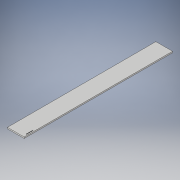
# Autodesk Inventor part: BBM
Saved by Autodesk Inventor 2019.4 (Build 234330000, 330)
## iProperties
Created: 2021-02-08
Part Number: BBM
Material: Generic
Document SubType Name: Modeling
Designer: caleb
Density: 1 g/cm^3
Appearance: Default
Author: caleb
Autodesk Inventor part; units mm, degrees
ref_plane "YZ Plane" through (0, 0, 0) normal (1, 0, 0) x (0, 1, 0)
ref_plane "XZ Plane" through (0, 0, 0) normal (0, 1, 0) x (-1, 0, 0)
ref_plane "XY Plane" through (0, 0, 0) normal (0, 0, 1) x (1, 0, 0)
sketch "Sketch1" plane through (0, 0, 0) normal (0, 1, 0) x (-1, 0, 0)
  line L0 (-2.5, 22.25) -> (2.5, 22.25)
  line L1 (2.5, 22.25) -> (2.5, -22.25)
  line L2 (2.5, -22.25) -> (-2.5, -22.25)
  line L3 (-2.5, -22.25) -> (-2.5, 22.25)
  line L4 (-2.5, 22.25) -> (2.5, -22.25) construction
  line L5 (2.5, 22.25) -> (-2.5, -22.25) construction
  point P0 (0, 0)
  dimension "d0" = 5
  dimension "d1" = 44.5
  constraints: 12 end point, 2 midpoint, 2 parallel, 1 horizontal, 1 perpendicular
  measures "d0" distance of L1.end L2.end
  measures "d1" distance of L0.end L1.end
extrude "Extrusion1" add sketch "Sketch1" along normal blind 0.4
sketch "Sketch2" plane through (0, 0.4, 0) normal (0, 1, 0) x (1, 0, 0)
  line L0 (2.07, -21.25) -> (2.2, -21.25)
  line L1 (2.2, -21.25) -> (2.2, -21.18)
  line L2 (2.2, -21.18) -> (2.07, -21.18)
  line L3 (2.07, -21.18) -> (2.07, -21.25)
  line L4 (2.07, -21.25) -> (2.2, -21.18) construction
  line L5 (2.2, -21.25) -> (2.07, -21.18) construction
  line L6 (-2.5, -22.25) -> (2.5, -22.25) projected
  line L7 (2.5, -22.25) -> (2.5, 22.25) projected
  line L8 (2.2, -21.08) -> (2.07, -21.08)
  line L9 (2.07, -21.08) -> (2.07, -21.15)
  line L10 (2.07, -21.15) -> (2.2, -21.15)
  line L11 (2.2, -21.15) -> (2.2, -21.08)
  line L12 (2.2, -20.98) -> (2.07, -20.98)
  line L13 (2.07, -20.98) -> (2.07, -21.05)
  line L14 (2.07, -21.05) -> (2.2, -21.05)
  line L15 (2.2, -21.05) -> (2.2, -20.98)
  line L16 (2.2, -20.88) -> (2.07, -20.88)
  line L17 (2.07, -20.88) -> (2.07, -20.95)
  line L18 (2.07, -20.95) -> (2.2, -20.95)
  line L19 (2.2, -20.95) -> (2.2, -20.88)
  line L20 (2.2, -20.78) -> (2.07, -20.78)
  line L21 (2.07, -20.78) -> (2.07, -20.85)
  line L22 (2.07, -20.85) -> (2.2, -20.85)
  line L23 (2.2, -20.85) -> (2.2, -20.78)
  line L24 (2.2, -20.68) -> (2.07, -20.68)
  line L25 (2.07, -20.68) -> (2.07, -20.75)
  line L26 (2.07, -20.75) -> (2.2, -20.75)
  line L27 (2.2, -20.75) -> (2.2, -20.68)
  line L28 (2.2, -20.58) -> (2.07, -20.58)
  line L29 (2.07, -20.58) -> (2.07, -20.65)
  line L30 (2.07, -20.65) -> (2.2, -20.65)
  line L31 (2.2, -20.65) -> (2.2, -20.58)
  line L32 (2.2, -20.48) -> (2.07, -20.48)
  line L33 (2.07, -20.48) -> (2.07, -20.55)
  line L34 (2.07, -20.55) -> (2.2, -20.55)
  line L35 (2.2, -20.55) -> (2.2, -20.48)
  line L36 (2.2, -20.38) -> (2.07, -20.38)
  line L37 (2.07, -20.38) -> (2.07, -20.45)
  line L38 (2.07, -20.45) -> (2.2, -20.45)
  line L39 (2.2, -20.45) -> (2.2, -20.38)
  line L40 (2.2, -20.28) -> (2.07, -20.28)
  line L41 (2.07, -20.28) -> (2.07, -20.35)
  line L42 (2.07, -20.35) -> (2.2, -20.35)
  line L43 (2.2, -20.35) -> (2.2, -20.28)
  line L44 (2.2, -20.18) -> (2.07, -20.18)
  line L45 (2.07, -20.18) -> (2.07, -20.25)
  line L46 (2.07, -20.25) -> (2.2, -20.25)
  line L47 (2.2, -20.25) -> (2.2, -20.18)
  line L48 (2.2, -20.08) -> (2.07, -20.08)
  line L49 (2.07, -20.08) -> (2.07, -20.15)
  line L50 (2.07, -20.15) -> (2.2, -20.15)
  line L51 (2.2, -20.15) -> (2.2, -20.08)
  line L52 (2.2, -19.98) -> (2.07, -19.98)
  line L53 (2.07, -19.98) -> (2.07, -20.05)
  line L54 (2.07, -20.05) -> (2.2, -20.05)
  line L55 (2.2, -20.05) -> (2.2, -19.98)
  line L56 (2.2, -19.88) -> (2.07, -19.88)
  line L57 (2.07, -19.88) -> (2.07, -19.95)
  line L58 (2.07, -19.95) -> (2.2, -19.95)
  line L59 (2.2, -19.95) -> (2.2, -19.88)
  line L60 (2.2, -19.78) -> (2.07, -19.78)
  line L61 (2.07, -19.78) -> (2.07, -19.85)
  line L62 (2.07, -19.85) -> (2.2, -19.85)
  line L63 (2.2, -19.85) -> (2.2, -19.78)
  line L64 (2.2, -19.68) -> (2.07, -19.68)
  line L65 (2.07, -19.68) -> (2.07, -19.75)
  line L66 (2.07, -19.75) -> (2.2, -19.75)
  line L67 (2.2, -19.75) -> (2.2, -19.68)
  line L68 (2.2, -19.58) -> (2.07, -19.58)
  line L69 (2.07, -19.58) -> (2.07, -19.65)
  line L70 (2.07, -19.65) -> (2.2, -19.65)
  line L71 (2.2, -19.65) -> (2.2, -19.58)
  line L72 (2.2, -19.48) -> (2.07, -19.48)
  line L73 (2.07, -19.48) -> (2.07, -19.55)
  line L74 (2.07, -19.55) -> (2.2, -19.55)
  line L75 (2.2, -19.55) -> (2.2, -19.48)
  line L76 (2.2, -19.38) -> (2.07, -19.38)
  line L77 (2.07, -19.38) -> (2.07, -19.45)
  line L78 (2.07, -19.45) -> (2.2, -19.45)
  line L79 (2.2, -19.45) -> (2.2, -19.38)
  line L80 (2.2, -19.28) -> (2.07, -19.28)
  line L81 (2.07, -19.28) -> (2.07, -19.35)
  line L82 (2.07, -19.35) -> (2.2, -19.35)
  line L83 (2.2, -19.35) -> (2.2, -19.28)
  point P0 (0, 0)
  point P1 (2.135, -21.215)
  point P2 (2.135, -21.115)
  point P3 (2.135, -21.015)
  point P4 (2.135, -20.915)
  point P5 (2.135, -20.815)
  point P6 (2.135, -20.715)
  point P7 (2.135, -20.615)
  point P8 (2.135, -20.515)
  point P9 (2.135, -20.415)
  point P10 (2.135, -20.315)
  point P11 (2.135, -20.215)
  point P12 (2.135, -20.115)
  point P13 (2.135, -20.015)
  point P14 (2.135, -19.915)
  point P15 (2.135, -19.815)
  point P16 (2.135, -19.715)
  point P17 (2.135, -19.615)
  point P18 (2.135, -19.515)
  point P19 (2.135, -19.415)
  point P20 (2.135, -19.315)
  dimension "d4" = 0.07
  dimension "d5" = 0.13
  dimension "d6" = 1
  dimension "d7" = 0.3
  dimension "d10" = 0.1
  constraints: 164 end point, 2 midpoint, 2 parallel, 1 horizontal, 1 perpendicular, 1 vertical, 171 other
  measures "d4" distance of L2.end L0.start
  measures "d5" distance of L1.end L2.end
  measures "d6" distance between parallel lines of L6 L0
  measures "d7" distance between parallel lines of L7 L1
  measures "d10" distance of point (2.135, -21.215) point (2.135, -21.115)
extrude "Extrusion2" add sketch "Sketch2" along normal blind 0.03
body "Solid1"
